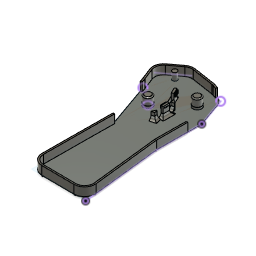
dualTriggerBase v36 (Autodesk Fusion 360 design; units mm, degrees)
Autodesk Fusion 360 part; units mm, degrees
note: some values were not read from the file. Chosen so that the rebuilt part matches the saved one: which pieces of a blend or face edit are solid. Set by a fixed rule: which sketch regions a step uses.
sketch "Sketch28" plane through (0, 0, 0) normal (0, 1, 0) x (1, 0, 0)
  line L0 (-35.000001, 0) -> (-28, -18)
  line L1 (-15, 15) -> (11, 11)
  line L2 (11, 11) -> (19.991799, 7.874299)
  line L3 (28.88127, -138.324499) -> (-14.117519, -138.001745)
  line L4 (-14.117519, -138.001745) -> (-13.525987, -59.195268)
  line L5 (-13.525987, -59.195268) -> (-28, -18)
  line L6 (28.88127, -138.324499) -> (29.770462, -19.862368)
  line L7 (29.770462, -19.862368) -> (19.991799, 7.874299)
  line L8 (-35.000001, 0) -> (-15, 15)
  line L9 (29.450629, -62.471964) -> (37.895462, -138.392161)
  line L10 (37.895462, -138.392161) -> (28.88127, -138.324499)
  dimension "d350" = 43
  constraint perpendicular L3 L6
  constraint perpendicular L6 L10
  constraint parallel L4 L6
  measures "d350" distance of L4 L6
extrude "Extrude27" add sketch "Sketch28" along normal blind 2
sketch "Sketch29" plane through (0, 2, 0) normal (0, 1, 0) x (-1, 0, 0)
  line L0 (35.000001, 0) -> (28, 18)
  line L1 (28, 18) -> (13.525987, 59.195268)
  line L2 (13.525987, 59.195268) -> (14.117519, 138.001745)
  line L3 (14.117519, 138.001745) -> (-37.895462, 138.392161)
  line L4 (-19.991799, -7.874299) -> (-11, -11)
  line L5 (-11, -11) -> (15, -15)
  circle A0 centre (-13.084148, 7.515386) radius 4
  circle A1 centre (-13.084148, 7.515386) radius 15
  circle A2 centre (19.92041, -4.133611) radius 2.25
  circle A3 centre (11.464587, 29.829591) radius 15
  circle A4 centre (11.464587, 29.829591) radius 4
  line L6 (-29.450629, 62.471964) -> (-29.770462, 19.862368)
  line L7 (-29.770462, 19.862368) -> (-19.991799, -7.874299)
  line L8 (15, -15) -> (35.000001, 0)
  line L9 (-37.895462, 138.392161) -> (-29.450629, 62.471964)
  line L10 (-13.084148, -34.372547) -> (-13.084148, 35.627453)
  line L11 (-13.084148, 7.515386) -> (6.965272, -4.060152)
  line L12 (11.464587, 7) -> (11.464587, 52.000001)
  line L13 (19.92041, -4.133611) -> (11.464587, 29.829591)
  point P0 (-13.084148, 7.515386)
  dimension "d199" = 8
  dimension "d200" = 4.5
  dimension "d202" = 8
  dimension "d203" = 35
  dimension "d204" = 30
  dimension "d205" = 30
  dimension "d340" = 35
  dimension "d341" = 60
  constraint concentric A3 A4
  constraint vertical L10
  constraint vertical L12
  measures "d199" diameter of A0
  measures "d200" diameter of A2
  measures "d202" diameter of A4
  measures "d204" diameter of A3
  measures "d205" diameter of A1
  measures "d341" angle of L10 L11
extrude "Extrude28" add sketch "Sketch29" along normal blind 7 contours A4 L12 L13 | A4 L12 L13 | A4 L12 | A0 L10 L11 | A0 L10 | A0 L10 L11 | A2 picked at (13.296687, 27.90191) picked at (12.002655, 27.220024) picked at (9.267444, 28.331604) picked at (-12.492418, 4.922848) picked at (-14.055667, 5.039997) picked at (-11.490146, 9.644724) picked at (19.294973, -3.405415)
sketch "Sketch30" plane through (0, 2, 0) normal (0, 1, 0) x (-1, 0, 0)
  circle A0 centre (-13.084148, 7.515386) radius 4
  circle A1 centre (19.92041, -4.133611) radius 2.25
  line L0 (35.000001, 0) -> (28, 18)
  line L1 (28, 18) -> (13.525987, 59.195268)
  line L2 (13.525987, 59.195268) -> (14.117519, 138.001745)
  line L3 (14.117519, 138.001745) -> (-37.895462, 138.392161)
  line L4 (-19.991799, -7.874299) -> (-11, -11)
  line L5 (-11, -11) -> (15, -15)
  circle A2 centre (11.464587, 29.829591) radius 4
  line L6 (-29.450629, 62.471964) -> (-29.770462, 19.862368)
  line L7 (-29.770462, 19.862368) -> (-19.991799, -7.874299)
  line L8 (15, -15) -> (35.000001, 0)
  line L9 (-37.895462, 138.392161) -> (-29.450629, 62.471964)
extrude "Extrude29" add 2 faces at (12.83959, 9, 8.469388) (-12.838324, 9, 30.766189) along direction (0, 1, 0) blind 2
sketch "Sketch31" plane through (0, 2, 0) normal (0, 1, 0) x (-1, 0, 0)
  circle A0 centre (11.464587, 29.829591) radius 4.15
  circle A1 centre (11.464587, 29.829591) radius 4
  circle A2 centre (-13.084148, 7.515386) radius 4
  circle A3 centre (-13.084148, 7.515386) radius 4.15
  dimension "d211" = 8.3
  dimension "d218" = 8.3
  constraint concentric A2 A3
  measures "d211" diameter of A0
  measures "d218" diameter of A3
extrude "Extrude30" add sketch "Sketch31" along normal blind 2 contours A0 | A1 | A3 picked at (14.599008, 32.456653) picked at (12.838324, 30.766189) picked at (-17.048004, 8.522313)
fillet "Fillet20" radius 1 2 edges at (-15.193896, 11, 31.276053) (9.354839, 11, 8.961848)
fillet "Fillet21" radius 10 7 edges at (-13.525987, 1, 59.195268) (-28, 1, 18) (11, 1, -11) (29.770462, 1, 19.862368) (-35.000001, 1, 0) (-15, 1, -15) (19.991799, 1, -7.874299)
fillet "Fillet22" radius 10 2 edges at (-14.117519, 1, 138.001745) (37.895462, 1, 138.392161)
sketch "Sketch32" plane through (0, 2, 0) normal (0, 1, 0) x (-1, 0, 0)
  arc A0 (-26.637031, 138.307654) -> (-36.650794, 127.202423) centre (-26.71209, 128.307935) ccw
  line L0 (-36.650794, 127.202423) -> (-29.450629, 62.471964)
  line L1 (-29.450629, 62.471964) -> (-29.757328, 21.612127)
  arc A1 (-29.757328, 21.612127) -> (-29.18866, 18.212116) centre (-19.75761, 21.537067) ccw
  line L2 (-29.18866, 18.212116) -> (-21.592397, -3.334286)
  arc A2 (-21.592397, -3.334286) -> (-15.444791, -9.454916) centre (-12.161347, -0.009335) ccw
  line L3 (-15.444791, -9.454916) -> (-11.861457, -10.700543)
  arc A3 (-11.861457, -10.700543) -> (-10.098585, -11.138679) centre (-8.578013, -1.254963) ccw
  line L4 (-10.098585, -11.138679) -> (10.843638, -14.36056)
  arc A4 (10.843638, -14.36056) -> (18.36421, -12.476843) centre (12.36421, -4.476843) ccw
  line L5 (18.36421, -12.476843) -> (28.929804, -4.552648)
  arc A5 (28.929804, -4.552648) -> (32.24985, 7.071815) centre (22.929804, 3.447352) ccw
  line L6 (32.24985, 7.071815) -> (28.059833, 17.846145)
  arc A6 (27.945279, 18.155747) -> (28.059833, 17.846145) centre (37.37988, 21.470607) ccw
  line L7 (27.945279, 18.155747) -> (14.104196, 57.549595)
  arc A7 (13.539079, 60.939514) -> (14.104196, 57.549595) centre (23.538798, 60.864455) ccw
  line L8 (13.539079, 60.939514) -> (14.04246, 128.002026)
  arc A8 (14.04246, 128.002026) -> (4.1178, 138.076804) centre (4.042741, 128.077086) ccw
  line L9 (4.1178, 138.076804) -> (-26.637031, 138.307654)
  circle A9 centre (-13.084148, 7.515386) radius 4.15
  circle A10 centre (11.464587, 29.829591) radius 4.15
  circle A11 centre (19.92041, -4.133611) radius 2.25
  line L10 (17.46421, -11.276843) -> (28.029804, -3.352648)
  arc A12 (28.029804, -3.352648) -> (30.851843, 6.528146) centre (22.929804, 3.447352) ccw
  line L11 (30.851843, 6.528146) -> (26.661826, 17.302475)
  arc A13 (26.530088, 17.658518) -> (26.661826, 17.302475) centre (37.37988, 21.470607) ccw
  line L12 (26.530088, 17.658518) -> (12.689006, 57.052366)
  arc A14 (12.039122, 60.950773) -> (12.689006, 57.052366) centre (23.538798, 60.864455) ccw
  line L13 (12.039122, 60.950773) -> (12.542502, 128.013285)
  arc A15 (12.542502, 128.013285) -> (4.106542, 136.576846) centre (4.042741, 128.077086) ccw
  line L14 (4.106542, 136.576846) -> (-26.648289, 136.807696)
  arc A16 (-26.648289, 136.807696) -> (-35.159988, 127.36825) centre (-26.71209, 128.307935) ccw
  line L15 (-35.159988, 127.36825) -> (-27.950005, 62.549518)
  line L16 (-27.950005, 62.549518) -> (-28.257371, 21.600868)
  arc A17 (-28.257371, 21.600868) -> (-27.774002, 18.710859) centre (-19.75761, 21.537067) ccw
  line L17 (-27.774002, 18.710859) -> (-20.177739, -2.835543)
  arc A18 (-20.177739, -2.835543) -> (-14.952274, -8.038078) centre (-12.161347, -0.009335) ccw
  line L18 (-14.952274, -8.038078) -> (-11.36894, -9.283706)
  arc A19 (-11.36894, -9.283706) -> (-9.870499, -9.656122) centre (-8.578013, -1.254963) ccw
  line L19 (-9.870499, -9.656122) -> (11.071724, -12.878002)
  arc A20 (11.071724, -12.878002) -> (17.46421, -11.276843) centre (12.36421, -4.476843) ccw
  line L20 (13.539079, 60.939514) -> (12.039122, 60.950773)
  line L21 (26.582297, 22.035003) -> (25.167106, 21.537774)
  line L22 (-15.444791, -9.454916) -> (-14.952274, -8.038078)
  line L23 (-28.171906, 32.986841) -> (-29.671864, 32.9981)
  dimension "d351" = -1.5
  constraint perpendicular L13 L20
  constraint perpendicular L12 L21
  constraint perpendicular L18 L22
  constraint perpendicular L1 L23
extrude "Extrude31" add sketch "Sketch32" along normal blind 8 contours A0 L0 L1 L8 A8 L9 L13 A15 L14 A16 L15 L16 L20 L23 | L3 A3 L4 A4 L5 A5 L6 A6 L7 L10 A12 L11 A13 L12 L18 A19 L19 A20 L21 L22 picked at (-30.853541, 84.129911) picked at (3.938926, -12.792414)
sketch "Sketch33" plane through (0, 2, 0) normal (0, 1, 0) x (-1, 0, 0)
  line L0 (-0.449636, 36.708271) -> (-3.347413, 35.931813)
  line L1 (-3.347413, 35.931813) -> (-4.123871, 38.829591)
  line L2 (-4.123871, 38.829591) -> (-1.226093, 39.606048)
  line L3 (-1.226093, 39.606048) -> (-0.449636, 36.708271)
  line L4 (27.204225, 29.829591) -> (-17.795776, 29.829591)
  line L5 (-13.084148, -9.033239) -> (-13.084148, 35.000001)
  line L6 (11.464587, 29.829591) -> (-4.123871, 38.829591)
  line L7 (-13.084148, 7.515386) -> (-2.759773, 22.260123)
  line L8 (-13.084148, 7.515386) -> (2.285263, 7.515386) construction
  line L9 (-2.759773, 22.260123) -> (-2.238828, 19.3057)
  line L10 (-2.238828, 19.3057) -> (-5.193251, 18.784755)
  line L11 (-5.193251, 18.784755) -> (-5.714196, 21.739179)
  line L12 (-5.714196, 21.739179) -> (-2.759773, 22.260123)
  point P0 (11.464587, 29.829591)
  point P1 (-13.084148, 7.515386)
  dimension "d237" = 3
  dimension "d244" = 3
  dimension "d301" = 30
  dimension "d302" = 18
  dimension "d303" = 18
  dimension "d304" = 55
  dimension "d305" = 3
  dimension "d306" = 3
  constraint horizontal L4
  constraint perpendicular L4 L5
  constraint perpendicular L0 L1
  constraint perpendicular L2 L3
  constraint perpendicular L1 L2
  constraint horizontal L8
  constraint perpendicular L9 L10
  constraint parallel L9 L11
  constraint parallel L10 L12
  measures "d301" angle of L4 L6
  measures "d304" angle of L7 L8
extrude "Extrude32" add sketch "Sketch33" along normal blind 6
chamfer "Chamfer8" distance 2.5 angle 45 2 edges at (0.449636, 5, 36.708271) (5.193251, 5, 18.784755)
sketch "Sketch34" plane through (5, 2, 67.213471) normal (0, 1, 0) x (-1, 0, 0)
  line L0 (3.773907, -27.607423) -> (3.903316, -28.090386)
  line L1 (3.903316, -28.090386) -> (2.135549, -31.152248)
  line L2 (2.135549, -31.152248) -> (1.652586, -31.281658)
  line L3 (1.652586, -31.281658) -> (0.876129, -28.38388)
  line L4 (0.876129, -28.38388) -> (3.773907, -27.607423)
  circle A0 centre (16.464586, -37.38388) radius 4.15
  circle A1 centre (-8.084149, -59.698085) radius 4.15
  line L5 (0.964586, -34.38388) -> (-1.035414, -34.38388)
  line L6 (-1.035414, -34.38388) -> (-1.035414, -40.38388)
  line L7 (-1.035414, -40.38388) -> (0.964586, -40.38388)
  line L8 (0.964586, -40.38388) -> (0.964586, -34.38388)
  line L9 (-0.714196, -45.474293) -> (2.240227, -44.953348)
  line L10 (2.240227, -44.953348) -> (2.761172, -47.907771)
  line L11 (2.761172, -47.907771) -> (2.268768, -47.994595)
  line L12 (2.268768, -47.994595) -> (-0.627372, -45.966696)
  line L13 (-0.627372, -45.966696) -> (-0.714196, -45.474293)
  line L14 (16.464586, -37.38388) -> (-1.035414, -37.38388)
  line L15 (-8.084149, -59.698085) -> (2.240227, -44.953348)
  line L16 (-8.084149, -59.698085) -> (7.776238, -52.302265)
  line L17 (9.044092, -55.021189) -> (7.231477, -55.866425)
  line L18 (7.231477, -55.866425) -> (4.695767, -50.428578)
  line L19 (4.695767, -50.428578) -> (6.508383, -49.583342)
  line L20 (6.508383, -49.583342) -> (9.044092, -55.021189)
  line L21 (9.044092, -55.021189) -> (4.695767, -50.428578) construction
  line L22 (7.231477, -55.866425) -> (6.508383, -49.583342) construction
  circle A2 centre (24.92041, -71.347082) radius 2.25
  line L23 (-9.952275, -75.25155) -> (-6.36894, -76.497177)
  arc A3 (-6.36894, -76.497177) -> (-4.870499, -76.869593) centre (-3.578013, -68.468434) ccw
  line L24 (-4.870499, -76.869593) -> (16.071724, -80.091473)
  arc A4 (16.071724, -80.091473) -> (22.46421, -78.490314) centre (17.36421, -71.690314) ccw
  line L25 (22.46421, -78.490314) -> (33.029803, -70.566119)
  arc A5 (33.029803, -70.566119) -> (35.851843, -60.685326) centre (27.929803, -63.766119) ccw
  line L26 (35.851843, -60.685326) -> (31.661826, -49.910996)
  arc A6 (31.530088, -49.554953) -> (31.661826, -49.910996) centre (42.37988, -45.742864) ccw
  line L27 (31.530088, -49.554953) -> (30.167106, -45.675697)
  line L28 (30.167106, -45.675697) -> (31.582296, -45.178468)
  line L29 (31.582296, -45.178468) -> (19.104196, -9.663876)
  arc A7 (18.539079, -6.273957) -> (19.104196, -9.663876) centre (28.538797, -6.349016) ccw
  line L30 (-24.671864, -34.215371) -> (-24.757329, -45.601344)
  arc A8 (-24.757329, -45.601344) -> (-24.18866, -49.001355) centre (-14.75761, -45.676404) ccw
  line L31 (-24.18866, -49.001355) -> (-16.592397, -70.547757)
  arc A9 (-16.592397, -70.547757) -> (-10.444791, -76.668387) centre (-7.161347, -67.222806) ccw
  line L32 (-10.444791, -76.668387) -> (-9.952275, -75.25155)
  line L33 (-23.171906, -34.22663) -> (-24.671864, -34.215371)
  line L34 (18.539079, -6.273957) -> (17.039121, -6.262698)
  line L35 (17.039121, -6.262698) -> (17.542502, 60.799814)
  arc A10 (17.542502, 60.799814) -> (9.106541, 69.363375) centre (9.042741, 60.863614) ccw
  line L36 (9.106541, 69.363375) -> (-21.64829, 69.594225)
  arc A11 (-21.64829, 69.594225) -> (-30.159989, 60.154779) centre (-21.71209, 61.094464) ccw
  line L37 (-30.159989, 60.154779) -> (-22.950005, -4.663953)
  line L38 (-22.950005, -4.663953) -> (-23.171906, -34.22663)
  point P0 (6.86993, -52.724884)
  dimension "d249" = 2
  dimension "d308" = 17.5
  dimension "d309" = 30
  dimension "d310" = 3
  dimension "d311" = 17.5
  dimension "d312" = 3
  dimension "d313" = 2
  constraint horizontal L5
  constraint vertical L6
  constraint horizontal L7
  constraint vertical L8
  constraint horizontal L14
  constraint perpendicular L17 L18
  constraint parallel L17 L19
  constraint parallel L18 L20
  measures "d309" angle of L15 L16
extrude "Extrude33" add sketch "Sketch34" along normal blind 9 contours L5 L6 L8 L14 | L6 L7 L8 L14 | L16 L18 L19 L20 | L16 L17 L18 L20 picked at (-0.368747, -35.38388) picked at (0.29792, -39.38388) picked at (6.145209, -51.959449) picked at (7.594651, -53.490319)
fillet "Fillet23" radius 3 10 edges at (6.035413, 2, 29.829591) (5.035413, 2, 32.829591) (2.674982, 2, 39.217819) (3.735642, 2, 37.380702) (4.236984, 2, 21.999651) (2.4993, 2, 20.782911) (5.035413, 2, 26.829591) (-0.602075, 2, 17.207511) (-2.776238, 2, 14.911206) (-3.137785, 2, 11.769664)
sketch "Sketch35" plane through (4.035413, 0, 0) normal (-1, 0, 0) x (0, 0, 1)
  line L0 (25.081473, 2) -> (35.747464, 2)
  line L1 (35.747464, 2) -> (35.747464, 2.001124)
  line L2 (32.829591, 5) -> (32.829591, 11)
  line L3 (32.829591, 11) -> (26.829591, 11)
  line L4 (26.829591, 11) -> (26.829591, 5)
  line L5 (27.779591, 8.4) -> (27.779591, 10)
  circle A0 centre (28.329591, 9.2) radius 0.5
  line L6 (31.879591, 8.4) -> (27.779591, 8.4)
  line L7 (27.779591, 10) -> (31.879591, 10)
  circle A1 centre (31.329591, 9.2) radius 0.5
  circle A2 centre (29.829591, 9.2) radius 0.5
  line L8 (31.879591, 10) -> (31.879591, 8.4)
  arc A3 (32.829591, 5) -> (35.747464, 2.001124) centre (35.829591, 5) ccw
  arc A4 (24.450741, 2.065009) -> (26.829591, 5) centre (23.829591, 5) ccw
  ellipse E0 centre (25.081473, 5) end of major axis (22.035193, 5) minor radius 3 (24.450741, 2.065009) -> (25.081473, 2) ccw
  point P0 (31.879591, 9.2)
  point P1 (29.829591, 10)
  dimension "d113" = 4.1
  dimension "d114" = 1.6
  dimension "d116" = 1
  dimension "d117" = 1
  dimension "d118" = 1.5
  dimension "d259" = 1.5
  dimension "d292" = 3
  dimension "d314" = 1
  constraint horizontal L7
  constraint vertical L8
  constraint horizontal L6
  constraint vertical L5
  measures "d116" diameter of A2
  measures "d117" diameter of A0
  measures "d314" distance of L3 L7
extrude "Extrude34" cut sketch "Sketch35" against normal blind 3 contours A0 | A1 | A2 picked at (28.066414, 9.379431) picked at (31.066414, 9.379431) picked at (29.566414, 9.379431)
sketch "Sketch36" plane through (4.035413, 0, 0) normal (-1, 0, 0) x (0, 0, 1)
  circle A0 centre (28.329591, 9.2) radius 0.5
  circle A1 centre (29.829591, 9.2) radius 0.5
  circle A2 centre (31.329591, 9.2) radius 0.5
  line L0 (25.081473, 2) -> (35.747464, 2)
  line L1 (35.747464, 2) -> (35.747464, 2.001124)
  line L2 (32.829591, 5) -> (32.829591, 11)
  line L3 (32.829591, 11) -> (26.829591, 11)
  line L4 (26.829591, 11) -> (26.829591, 5)
  line L5 (27.729591, 10.05) -> (31.929591, 10.05)
  line L6 (31.929591, 10.05) -> (31.929591, 8.35)
  line L7 (31.929591, 8.35) -> (27.729591, 8.35)
  line L8 (27.729591, 8.35) -> (27.729591, 10.05)
  line L9 (32.429591, 10.55) -> (27.229591, 10.55)
  line L10 (27.229591, 10.55) -> (27.229591, 7.85)
  line L11 (27.229591, 7.85) -> (32.429591, 7.85)
  line L12 (32.429591, 7.85) -> (32.429591, 10.55)
  line L13 (32.429591, 10.55) -> (27.229591, 7.85) construction
  line L14 (27.229591, 10.55) -> (32.429591, 7.85) construction
  arc A3 (32.829591, 5) -> (35.747464, 2.001124) centre (35.829591, 5) ccw
  arc A4 (24.450741, 2.065009) -> (26.829591, 5) centre (23.829591, 5) ccw
  ellipse E0 centre (25.081473, 5) end of major axis (22.035193, 5) minor radius 3 (24.450741, 2.065009) -> (25.081473, 2) ccw
  point P0 (31.929591, 9.2)
  point P1 (29.829591, 10.05)
  point P2 (29.829591, 9.2)
  dimension "d262" = 4.2
  dimension "d263" = 1.7
  dimension "d264" = 5.2
  dimension "d265" = 2.7
  constraint horizontal L5
  constraint vertical L6
  constraint horizontal L7
  constraint vertical L8
  constraint horizontal L9
  constraint perpendicular L9 L10
  constraint parallel L9 L11
  constraint parallel L10 L12
extrude "Extrude35" add sketch "Sketch36" along normal blind 1 contours L9 L10 L11 L12 picked at (29.129591, 8.016667)
fillet "Fillet24" radius 0.3 4 edges at (4.035413, 10.55, 29.829591) (4.035413, 9.2, 32.429591) (4.035413, 9.2, 27.229591) (4.035413, 7.85, 29.829591)
sketch "Sketch39" plane through (-6.179092, 0, 2.881358) normal (0.906308, 0, -0.422618) x (-0.422618, 0, -0.906308)
  line L0 (-18.258727, 2) -> (-6.340853, 2)
  arc A0 (-9.340853, 5) -> (-6.340853, 2) centre (-6.340853, 5) ccw
  line L1 (-9.340853, 5) -> (-9.340853, 11)
  line L2 (-9.340853, 11) -> (-15.340853, 11)
  line L3 (-15.340853, 11) -> (-15.340853, 5)
  arc A1 (-18.258727, 2.001124) -> (-15.340853, 5) centre (-18.340853, 5) ccw
  line L4 (27.779591, 10) -> (31.879591, 10)
  line L5 (31.879591, 8.4) -> (27.779591, 8.4)
  circle A2 centre (29.829591, 9.2) radius 0.5
  circle A3 centre (28.329591, 9.2) radius 0.5
  line L6 (27.779591, 8.4) -> (27.779591, 10)
  line L7 (32.829591, 11) -> (26.829591, 11)
  line L8 (31.879591, 10) -> (31.879591, 8.4)
  circle A4 centre (31.329591, 9.2) radius 0.5
  line L9 (-14.440853, 10) -> (-10.240853, 10)
  line L10 (-10.240853, 10) -> (-10.240853, 8.3)
  line L11 (-10.240853, 8.3) -> (-14.440853, 8.3)
  line L12 (-14.440853, 8.3) -> (-14.440853, 10)
  circle A5 centre (-12.340853, 9.15) radius 0.5
  circle A6 centre (-13.840853, 9.15) radius 0.5
  circle A7 centre (-10.840853, 9.15) radius 0.5
  line L13 (-18.258727, 2.001124) -> (-18.258727, 2)
  point P0 (29.829591, 10)
  point P1 (31.879591, 9.2)
  point P2 (-12.340853, 10)
  point P3 (-12.340853, 11)
  point P4 (-10.240853, 9.15)
  dimension "d315" = 4.1
  dimension "d316" = 1.6
  dimension "d317" = 1
  dimension "d318" = 1
  dimension "d319" = 1.5
  dimension "d320" = 1.5
  dimension "d321" = 1
  dimension "d322" = 4.2
  dimension "d323" = 1.7
  dimension "d324" = 1
  dimension "d325" = 1
  dimension "d326" = 1
  dimension "d327" = 1
  dimension "d328" = 1.5
  dimension "d329" = 1.5
  constraint horizontal L4
  constraint vertical L8
  constraint horizontal L5
  constraint vertical L6
  constraint horizontal L9
  constraint vertical L10
  constraint horizontal L11
  constraint vertical L12
  measures "d317" diameter of A2
  measures "d318" diameter of A3
  measures "d321" distance of L4 L7
  measures "d324" distance of L2 L9
  measures "d325" diameter of A5
  measures "d326" diameter of A6
  measures "d327" diameter of A7
extrude "Extrude38" cut sketch "Sketch39" against normal blind 3 contours A5 | A6 | A7 picked at (-12.588992, 9.070344) picked at (-14.135238, 9.088494) picked at (-11.135238, 9.088494)
sketch "Sketch40" plane through (-6.179092, 0, 2.881358) normal (0.906308, 0, -0.422618) x (-0.422618, 0, -0.906308)
  circle A0 centre (-13.840853, 9.15) radius 0.5
  circle A1 centre (-12.340853, 9.15) radius 0.5
  circle A2 centre (-10.840853, 9.15) radius 0.5
  line L0 (-18.258727, 2) -> (-6.340853, 2)
  arc A3 (-9.340853, 5) -> (-6.340853, 2) centre (-6.340853, 5) ccw
  line L1 (-9.340853, 5) -> (-9.340853, 11)
  line L2 (-9.340853, 11) -> (-15.340853, 11)
  line L3 (-15.340853, 11) -> (-15.340853, 5)
  arc A4 (-18.258727, 2.001124) -> (-15.340853, 5) centre (-18.340853, 5) ccw
  line L4 (-10.240853, 10) -> (-14.440853, 10)
  line L5 (-14.440853, 10) -> (-14.440853, 8.3)
  line L6 (-14.440853, 8.3) -> (-10.240853, 8.3)
  line L7 (-10.240853, 8.3) -> (-10.240853, 10)
  line L8 (-10.240853, 10) -> (-14.440853, 8.3) construction
  line L9 (-14.440853, 10) -> (-10.240853, 8.3) construction
  line L10 (-9.740853, 10.5) -> (-14.940853, 10.5)
  line L11 (-14.940853, 10.5) -> (-14.940853, 7.8)
  line L12 (-14.940853, 7.8) -> (-9.740853, 7.8)
  line L13 (-9.740853, 7.8) -> (-9.740853, 10.5)
  line L14 (-9.740853, 10.5) -> (-14.940853, 7.8) construction
  line L15 (-14.940853, 10.5) -> (-9.740853, 7.8) construction
  line L16 (-18.258727, 2.001124) -> (-18.258727, 2)
  point P0 (-12.340853, 9.15)
  point P1 (-12.340853, 9.15)
  dimension "d332" = 4.2
  dimension "d333" = 1.7
  dimension "d334" = 5.2
  dimension "d335" = 2.7
  constraint horizontal L4
  constraint perpendicular L4 L5
  constraint parallel L4 L6
  constraint parallel L5 L7
  constraint horizontal L10
  constraint perpendicular L10 L11
  constraint parallel L10 L12
  constraint parallel L11 L13
extrude "Extrude39" add sketch "Sketch40" along normal blind 1 contours L10 L11 L12 L13 picked at (-11.640853, 7.966667)
fillet "Fillet27" radius 0.4 4 edges at (-0.963622, 10.5, 14.065969) (-2.06243, 9.15, 11.709569) (-0.963622, 7.8, 14.065969) (0.135185, 9.15, 16.42237)
fillet "Fillet28" radius 2 19 edges at (29.603979, 0, 42.042045) (33.050712, 0, 94.837193) (34.138691, 0, 135.00462) (11.259615, 0, 138.192229) (-11.166685, 0, 135.094879) (-13.790769, 0, 94.47077) (-13.67492, 0, 59.220096) (-21.024737, 0, 37.852671) (-28.001278, 0, 18.000473) (-30.154842, 0, 12.45898) (-32.545311, 0, 0.70108) (-23.647007, 0, -8.514745) (-14.793905, 0, -14.177182) (-0.372527, 0, -12.74962) (10.98999, 0, -10.959723) (13.653124, 0, -10.077729) (19.216849, 0, -7.095934) (25.390528, 0, 7.438915) (29.620607, 0, 19.887433)
equation "d259 = d118"
equation "d320 = d118"
